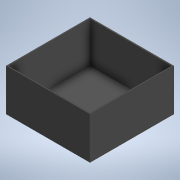
# Autodesk Inventor part: techo
Saved by Autodesk Inventor 2020 (Build 240168000, 168)
## iProperties
Created: 2021-10-17
Part Number: techo
Material: Genérico
Document SubType Name: Modeling
Designer: DANIEL
Density: 1 g/cm^3
Appearance: Genérico
Author: DANIEL
Autodesk Inventor part; units mm, degrees
ref_plane "YZ Plane" through (0, 0, 0) normal (1, 0, 0) x (0, 1, 0)
ref_plane "XZ Plane" through (0, 0, 0) normal (0, 1, 0) x (-1, 0, 0)
ref_plane "XY Plane" through (0, 0, 0) normal (0, 0, 1) x (1, 0, 0)
sketch "Boceto1" plane through (0, 0, 0) normal (0, 1, 0) x (-1, 0, 0)
  line L0 (200, 200) -> (-200, 200)
  line L1 (-200, 200) -> (-200, -200)
  line L2 (-200, -200) -> (200, -200)
  line L3 (200, -200) -> (200, 200)
  line L4 (195, 195) -> (-195, 195)
  line L5 (-195, 195) -> (-195, -195)
  line L6 (-195, -195) -> (195, -195)
  line L7 (195, -195) -> (195, 195)
  point P0 (0, 0)
  dimension "L" = 400
  dimension "d1" = 400
  dimension "d2" = 200
  dimension "d3" = 200
  dimension "d4" = 390
  dimension "d5" = 390
  dimension "d6" = 195
  dimension "d7" = 195
  constraints: 16 end point, 4 parallel, 2 horizontal, 2 perpendicular
  measures "L" distance of L0.start L0.end
  measures "d1" distance of L0.end L1.end
  measures "d2" distance from line of L2 point (0, 0)
  measures "d3" distance from line of point (0, 0) L1
  measures "d4" distance between parallel lines of L6 L4
  measures "d5" distance between parallel lines of L5 L7
  measures "d6" distance from line of L7 point (0, 0)
  measures "d7" distance from line of L4 point (0, 0)
extrude "Extrusión1" add sketch "Boceto1" along normal blind 200
sketch "Boceto2" plane through (0, 0, 0) normal (0, -1, 0) x (1, 0, 0)
  line L0 (195, 195) -> (-195, 195) projected
  line L1 (-195, -195) -> (195, -195) projected
  line L2 (195, 195) -> (-195, 195)
  line L3 (-195, 195) -> (-195, -195)
  line L4 (-195, -195) -> (195, -195)
  line L5 (195, -195) -> (195, 195)
  point P0 (0, 0)
  point P1 (195, -195)
  constraints: 8 end point, 2 parallel, 1 horizontal, 1 perpendicular
extrude "Extrusión2" add sketch "Boceto2" against normal blind 5
equation "\"d1\" = L"
equation "\"d2\" = 0.5 * L"
equation "\"d3\" = 0.5 * L"
